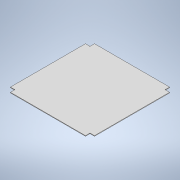
# Autodesk Inventor part: Acrylicsheet
Saved by Autodesk Inventor 2020.2 (Build 242310000, 310)
## iProperties
Created: 2020-07-30
Part Number: Acrylicsheet
Material: Generic
Document SubType Name: Modeling
Designer: JK
Density: 1 g/cm^3
Appearance: Default
Author: JK
Autodesk Inventor part; units mm, degrees
ref_plane "YZ Plane" through (0, 0, 0) normal (1, 0, 0) x (0, 1, 0)
ref_plane "XZ Plane" through (0, 0, 0) normal (0, 1, 0) x (-1, 0, 0)
ref_plane "XY Plane" through (0, 0, 0) normal (0, 0, 1) x (1, 0, 0)
sketch "Sketch1" plane through (0, 0, 0) normal (0, 1, 0) x (-1, 0, 0)
  line L0 (-280, 280) -> (280, 280)
  line L1 (280, 280) -> (280, -280)
  line L2 (280, -280) -> (-280, -280)
  line L3 (-280, -280) -> (-280, 280)
  line L4 (-280, 280) -> (280, -280) construction
  line L5 (280, 280) -> (-280, -280) construction
  point P0 (0, 0)
  dimension "d0" = 560
  dimension "d1" = 560
  constraints: 12 end point, 2 midpoint, 2 parallel, 1 horizontal, 1 perpendicular
  measures "d0" distance of L0.end L1.end
  measures "d1" distance of L1.end L2.end
extrude "Extrusion1" add sketch "Sketch1" along normal blind 4
sketch "Sketch2" plane through (0, 4, 0) normal (0, 1, 0) x (1, 0, 0)
  line L0 (-280, 280) -> (-280, -280) projected
  line L1 (-280, -280) -> (-250, -280)
  line L2 (-250, -280) -> (-250, -250)
  line L3 (-250, -250) -> (-280, -250)
  line L4 (-280, -250) -> (-280, -280)
  line L5 (-280, 280) -> (-250, 280)
  line L6 (-250, 280) -> (-250, 250)
  line L7 (-250, 250) -> (-280, 250)
  line L8 (-280, 250) -> (-280, 280)
  line L9 (280, -280) -> (280, 280) projected
  line L10 (280, 280) -> (250, 280)
  line L11 (250, 280) -> (250, 250)
  line L12 (250, 250) -> (280, 250)
  line L13 (280, 250) -> (280, 280)
  line L14 (280, -280) -> (250, -280)
  line L15 (250, -280) -> (250, -250)
  line L16 (250, -250) -> (280, -250)
  line L17 (280, -250) -> (280, -280)
  point P0 (0, 0)
  dimension "d4" = 30
  dimension "d5" = 30
  dimension "d6" = 30
  dimension "d7" = 30
  dimension "d8" = 30
  dimension "d9" = 30
  constraints: 32 end point, 8 parallel, 4 horizontal, 4 perpendicular, 2 equal length
  measures "d4" distance of L2.end L3.end
  measures "d5" distance of L1.end L2.end
  measures "d6" distance between parallel lines of L8 L6
  measures "d7" distance between parallel lines of L5 L7
  measures "d8" distance between parallel lines of L13 L11
  measures "d9" distance between parallel lines of L10 L12
extrude "Extrusion2" cut sketch "Sketch2" against normal blind 10
body "Solid1"
